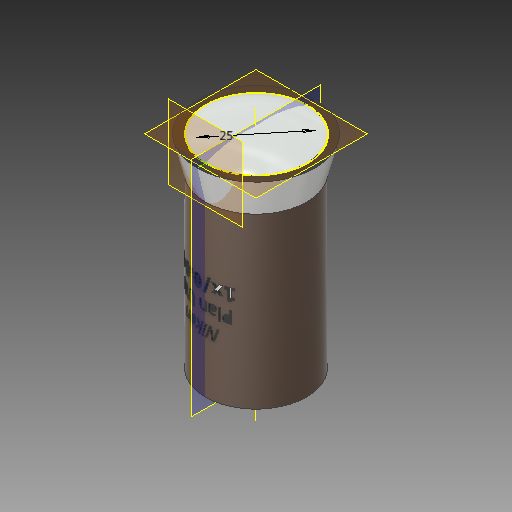
# Autodesk Inventor part: NikonObjective1x
Saved by Autodesk Inventor 2017 (Build 210142000, 142)
## iProperties
Created: 2016-05-20
Part Number: NikonObjective1x
Material: Generic
Document SubType Name: Modeling
Designer: symvoulidis
Density: 1 g/cm^3
Appearance: Smooth - Black
Author: symvoulidis
Autodesk Inventor part; units mm, degrees
ref_plane "YZ Plane" through (0, 0, 0) normal (1, 0, 0) x (0, 1, 0)
ref_plane "XZ Plane" through (0, 0, 0) normal (0, 1, 0) x (-1, 0, 0)
ref_plane "XY Plane" through (0, 0, 0) normal (0, 0, 1) x (1, 0, 0)
sketch "Sketch1" plane through (0, 0, 0) normal (0, 1, 0) x (-1, 0, 0)
  circle A0 centre (0, 0) radius 15
  dimension "d0" = 30
  constraints: 1 centre point, 1 coincident
  measures "d0" diameter of A0
extrude "Extrusion1" add sketch "Sketch1" along normal blind 50
ref_plane "Work Plane1" through (0, 60, 0) normal (0, 1, 0) x (1, 0, 0)
sketch "Sketch2" plane through (0, 60, 0) normal (0, 1, 0) x (1, 0, 0)
  circle A0 centre (0, 0) radius 15 projected
  circle A1 centre (0, 0) radius 12.5
  point P0 (0, -15)
  dimension "d11" = 25
  constraints: 1 centre point, 1 coincident, 1 vertical alignment, 1 other
  measures "d11" diameter of A1
sketch "Sketch3" plane through (0, 60, 0) normal (0, 1, 0) x (1, 0, 0)
  circle A0 centre (0, 0) radius 17.5
  dimension "d4" = 35
  constraints: 1 centre point, 1 coincident
  measures "d4" diameter of A0
loft "Loft1" add profiles "Sketch3" section 2 edges at (15, 50, 0)
ref_plane "Work Plane2" through (0, 60, 15) normal (0, 0, 1) x (1, 0, 0)
sketch "Sketch4" plane through (0, 60, 15) normal (0, 0, 1) x (1, 0, 0)
  line L0 (8.3999, -44.7935) -> (-12.4534, -44.7935) construction
  line L1 (-12.4534, -44.7935) -> (-12.4534, -35.0395) construction
  line L2 (-12.4534, -35.0395) -> (8.3999, -35.0395) construction
  line L3 (8.3999, -35.0395) -> (8.3999, -44.7935) construction
  line L4 (1.1783, -41.1375) -> (1.7002, -41.1375)
  line L5 (1.7002, -41.1375) -> (2.222, -44.1553)
  line L6 (2.222, -44.1553) -> (3.2488, -41.1375)
  line L7 (3.2488, -41.1375) -> (3.6827, -41.1375)
  line L8 (3.6827, -41.1375) -> (2.4943, -44.6375)
  line L9 (2.4943, -44.6375) -> (1.8335, -44.6375)
  line L10 (1.8335, -44.6375) -> (1.3655, -41.8664)
  line L11 (1.3655, -41.8664) -> (0.4238, -44.6375)
  line L12 (0.4238, -44.6375) -> (-0.0101, -44.6375)
  line L13 (-0.0101, -44.6375) -> (1.1783, -41.1375)
  line L14 (0.0523, -41.1375) -> (0.4947, -41.1375)
  line L15 (0.4947, -41.1375) -> (-0.3987, -43.7639)
  line L16 (-0.3987, -43.7639) -> (-0.8412, -43.7639)
  line L17 (-0.8412, -43.7639) -> (0.0523, -41.1375)
  line L18 (-1.0199, -44.2007) -> (-0.5178, -44.2007)
  line L19 (-0.5178, -44.2007) -> (-0.6738, -44.6602)
  line L20 (-0.6738, -44.6602) -> (-1.1759, -44.6602)
  line L21 (-1.1759, -44.6602) -> (-1.0199, -44.2007)
  line L22 (-2.7727, -41.1375) -> (-2.1912, -41.1375)
  line L23 (-2.1912, -41.1375) -> (-1.6467, -42.4053)
  line L24 (-1.6467, -42.4053) -> (-1.4141, -42.2352)
  line L25 (-1.4141, -42.2352) -> (-1.0397, -41.1375)
  line L26 (-1.0397, -41.1375) -> (-0.5972, -41.1375)
  line L27 (-0.5972, -41.1375) -> (-1.8395, -44.7935)
  line L28 (-1.8395, -44.7935) -> (-2.282, -44.7935)
  line L29 (-2.282, -44.7935) -> (-1.5559, -42.6549)
  line L30 (-1.5559, -42.6549) -> (-2.9712, -43.7639)
  line L31 (-2.9712, -43.7639) -> (-3.5215, -43.7639)
  line L32 (-3.5215, -43.7639) -> (-2.0721, -42.6663)
  line L33 (-2.0721, -42.6663) -> (-2.7727, -41.1375)
  spline S0 degree 2 poles (-5.5977, -42.4507) (-5.3736, -41.787) (-4.4887, -41.0638) (-3.9554, -41.0638) knots 0 0 0 1 2 2 2
  spline S1 degree 2 poles (-3.9554, -41.0638) (-3.408, -41.0638) (-3.0365, -41.8097) (-3.252, -42.4507) knots 0 0 0 1 2 2 2
  spline S2 degree 2 poles (-3.252, -42.4507) (-3.4761, -43.1087) (-4.3695, -43.8377) (-4.8999, -43.8377) knots 0 0 0 1 2 2 2
  spline S3 degree 2 poles (-4.8999, -43.8377) (-5.4303, -43.8377) (-5.8217, -43.1116) (-5.5977, -42.4507) knots 0 0 0 1 2 2 2
  spline S4 degree 2 poles (-5.141, -42.4507) (-5.314, -42.9613) (-5.1126, -43.4576) (-4.7695, -43.4576) knots 0 0 0 1 2 2 2
  spline S5 degree 2 poles (-4.7695, -43.4576) (-4.4263, -43.4576) (-3.8817, -42.9613) (-3.7087, -42.4507) knots 0 0 0 1 2 2 2
  spline S6 degree 2 poles (-3.7087, -42.4507) (-3.5413, -41.9544) (-3.7399, -41.4438) (-4.0859, -41.4438) knots 0 0 0 1 2 2 2
  spline S7 degree 2 poles (-4.0859, -41.4438) (-4.4263, -41.4438) (-4.9708, -41.9459) (-5.141, -42.4507) knots 0 0 0 1 2 2 2
  line L34 (-7.6682, -41.1375) -> (-7.2257, -41.1375)
  line L35 (-7.2257, -41.1375) -> (-7.7334, -42.6351)
  spline S8 degree 2 poles (-7.7334, -42.6351) (-7.7958, -42.8166) (-7.8667, -43.1286) (-7.8497, -43.2222) knots 0 0 0 1 2 2 2
  spline S9 degree 2 poles (-7.8497, -43.2222) (-7.8298, -43.3215) (-7.671, -43.4179) (-7.5036, -43.4179) knots 0 0 0 1 2 2 2
  spline S10 degree 2 poles (-7.5036, -43.4179) (-7.3391, -43.4179) (-6.9307, -43.242) (-6.7152, -43.1002) knots 0 0 0 1 2 2 2
  line L36 (-6.7152, -43.1002) -> (-6.0486, -41.1375)
  line L37 (-6.0486, -41.1375) -> (-5.6062, -41.1375)
  line L38 (-5.6062, -41.1375) -> (-6.4996, -43.7639)
  line L39 (-6.4996, -43.7639) -> (-6.9421, -43.7639)
  line L40 (-6.9421, -43.7639) -> (-6.8428, -43.4718)
  spline S11 degree 2 poles (-6.8428, -43.4718) (-7.1009, -43.6505) (-7.549, -43.8377) (-7.7618, -43.8377) knots 0 0 0 1 2 2 2
  spline S12 degree 2 poles (-7.7618, -43.8377) (-8.1503, -43.8377) (-8.4113, -43.3271) (-8.2468, -42.8421) knots 0 0 0 1 2 2 2
  line L41 (-8.2468, -42.8421) -> (-7.6682, -41.1375)
  spline S13 degree 2 poles (4.389, -37.8197) (4.389, -37.5928) (4.5506, -37.1844) (4.6953, -37.0426) knots 0 0 0 1 2 2 2
  spline S14 degree 2 poles (4.6953, -37.0426) (4.8768, -36.8639) (5.3675, -36.6796) (5.7419, -36.6796) knots 0 0 0 1 2 2 2
  line L42 (5.7419, -36.6796) -> (6.1361, -36.6796)
  line L43 (6.1361, -36.6796) -> (6.1361, -35.3749)
  line L44 (6.1361, -35.3749) -> (6.6013, -35.3749)
  line L45 (6.6013, -35.3749) -> (6.6013, -38.8749)
  line L46 (6.6013, -38.8749) -> (5.722, -38.8749)
  spline S15 degree 2 poles (5.722, -38.8749) (5.41, -38.8749) (4.9733, -38.7727) (4.8059, -38.6565) knots 0 0 0 1 2 2 2
  spline S16 degree 2 poles (4.8059, -38.6565) (4.6102, -38.5231) (4.389, -38.1119) (4.389, -37.8197) knots 0 0 0 1 2 2 2
  spline S17 degree 2 poles (4.874, -37.8056) (4.874, -37.9871) (4.9988, -38.2537) (5.1264, -38.3388) knots 0 0 0 1 2 2 2
  spline S18 degree 2 poles (5.1264, -38.3388) (5.237, -38.4125) (5.532, -38.4721) (5.7504, -38.4721) knots 0 0 0 1 2 2 2
  line L47 (5.7504, -38.4721) -> (6.1361, -38.4721)
  line L48 (6.1361, -38.4721) -> (6.1361, -37.0766)
  line L49 (6.1361, -37.0766) -> (5.8185, -37.0766)
  spline S19 degree 2 poles (5.8185, -37.0766) (5.5348, -37.0766) (5.186, -37.1674) (5.0725, -37.2865) knots 0 0 0 1 2 2 2
  spline S20 degree 2 poles (5.0725, -37.2865) (4.9676, -37.3915) (4.874, -37.6382) (4.874, -37.8056) knots 0 0 0 1 2 2 2
  line L50 (3.5296, -35.3749) -> (3.972, -35.3749)
  line L51 (3.972, -35.3749) -> (3.972, -39.0308)
  line L52 (3.972, -39.0308) -> (3.5296, -39.0308)
  line L53 (3.5296, -39.0308) -> (3.5296, -35.3749)
  spline S21 degree 2 poles (1.4165, -35.6528) (1.4704, -35.6131) (1.6519, -35.4713) (1.737, -35.4287) knots 0 0 0 1 2 2 2
  spline S22 degree 2 poles (1.737, -35.4287) (1.8533, -35.3663) (2.0717, -35.3011) (2.2703, -35.3011) knots 0 0 0 1 2 2 2
  spline S23 degree 2 poles (2.2703, -35.3011) (2.4319, -35.3011) (2.7241, -35.4231) (2.8347, -35.5337) knots 0 0 0 1 2 2 2
  spline S24 degree 2 poles (2.8347, -35.5337) (2.9396, -35.6415) (3.0673, -35.9591) (3.0673, -36.135) knots 0 0 0 1 2 2 2
  spline S25 degree 2 poles (3.0673, -36.135) (3.0673, -36.4073) (2.8375, -36.793) (2.5879, -36.9036) knots 0 0 0 1 2 2 2
  spline S26 degree 2 poles (2.5879, -36.9036) (2.3667, -37.0057) (1.7654, -37.0823) (1.4165, -37.1022) knots 0 0 0 1 2 2 2
  line L54 (1.4165, -37.1022) -> (1.4165, -37.1872)
  spline S27 degree 2 poles (1.4165, -37.1872) (1.4165, -37.3404) (1.5101, -37.5304) (1.5952, -37.5843) knots 0 0 0 1 2 2 2
  spline S28 degree 2 poles (1.5952, -37.5843) (1.6803, -37.6382) (1.9242, -37.6723) (2.0547, -37.6723) knots 0 0 0 1 2 2 2
  spline S29 degree 2 poles (2.0547, -37.6723) (2.2079, -37.6723) (2.622, -37.5815) (2.829, -37.4936) knots 0 0 0 1 2 2 2
  line L55 (2.829, -37.4936) -> (2.8545, -37.4936)
  line L56 (2.8545, -37.4936) -> (2.8545, -37.9445)
  spline S30 degree 2 poles (2.8545, -37.9445) (2.7326, -37.9786) (2.2759, -38.0637) (2.0519, -38.0637) knots 0 0 0 1 2 2 2
  spline S31 degree 2 poles (2.0519, -38.0637) (1.7796, -38.0637) (1.408, -37.9786) (1.2605, -37.868) knots 0 0 0 1 2 2 2
  spline S32 degree 2 poles (1.2605, -37.868) (1.1159, -37.7602) (0.9741, -37.417) (0.9741, -37.1702) knots 0 0 0 1 2 2 2
  line L57 (0.9741, -37.1702) -> (0.9741, -35.3749)
  line L58 (0.9741, -35.3749) -> (1.4165, -35.3749)
  line L59 (1.4165, -35.3749) -> (1.4165, -35.6528)
  line L60 (1.4165, -36.0215) -> (1.4165, -36.7505)
  spline S33 degree 2 poles (1.4165, -36.7505) (1.5754, -36.7363) (2.0547, -36.6881) (2.205, -36.6427) knots 0 0 0 1 2 2 2
  spline S34 degree 2 poles (2.205, -36.6427) (2.3809, -36.5888) (2.6106, -36.3647) (2.6106, -36.1662) knots 0 0 0 1 2 2 2
  spline S35 degree 2 poles (2.6106, -36.1662) (2.6106, -35.9393) (2.3553, -35.7095) (2.1114, -35.7095) knots 0 0 0 1 2 2 2
  spline S36 degree 2 poles (2.1114, -35.7095) (1.9044, -35.7095) (1.564, -35.8882) (1.4165, -36.0215) knots 0 0 0 1 2 2 2
  line L61 (-1.7091, -35.3749) -> (-1.2666, -35.3749)
  line L62 (-1.2666, -35.3749) -> (-1.2666, -36.8724)
  spline S37 degree 2 poles (-1.2666, -36.8724) (-1.2666, -37.0539) (-1.2326, -37.3659) (-1.1815, -37.4595) knots 0 0 0 1 2 2 2
  spline S38 degree 2 poles (-1.1815, -37.4595) (-1.1276, -37.5588) (-0.9348, -37.6552) (-0.7703, -37.6552) knots 0 0 0 1 2 2 2
  spline S39 degree 2 poles (-0.7703, -37.6552) (-0.6058, -37.6552) (-0.2569, -37.4794) (-0.0895, -37.3376) knots 0 0 0 1 2 2 2
  line L63 (-0.0895, -37.3376) -> (-0.0895, -35.3749)
  line L64 (-0.0895, -35.3749) -> (0.3529, -35.3749)
  line L65 (0.3529, -35.3749) -> (0.3529, -38.0013)
  line L66 (0.3529, -38.0013) -> (-0.0895, -38.0013)
  line L67 (-0.0895, -38.0013) -> (-0.0895, -37.7091)
  spline S40 degree 2 poles (-0.0895, -37.7091) (-0.2881, -37.8878) (-0.671, -38.075) (-0.8865, -38.075) knots 0 0 0 1 2 2 2
  spline S41 degree 2 poles (-0.8865, -38.075) (-1.2723, -38.075) (-1.7091, -37.5645) (-1.7091, -37.0795) knots 0 0 0 1 2 2 2
  line L68 (-1.7091, -37.0795) -> (-1.7091, -35.3749)
  spline S42 degree 2 poles (-5.09, -35.3011) (-4.7808, -35.3011) (-4.3213, -35.4628) (-4.1596, -35.6244) knots 0 0 0 1 2 2 2
  spline S43 degree 2 poles (-4.1596, -35.6244) (-3.9753, -35.806) (-3.825, -36.3165) (-3.825, -36.6909) knots 0 0 0 1 2 2 2
  line L69 (-3.825, -36.6909) -> (-3.825, -38.8749)
  line L70 (-3.825, -38.8749) -> (-4.2901, -38.8749)
  line L71 (-4.2901, -38.8749) -> (-4.2901, -36.6909)
  spline S44 degree 2 poles (-4.2901, -36.6909) (-4.2901, -36.447) (-4.3525, -36.118) (-4.4404, -35.9847) knots 0 0 0 1 2 2 2
  spline S45 degree 2 poles (-4.4404, -35.9847) (-4.534, -35.8428) (-4.8574, -35.6982) (-5.09, -35.6982) knots 0 0 0 1 2 2 2
  spline S46 degree 2 poles (-5.09, -35.6982) (-5.3083, -35.6982) (-5.6487, -35.8428) (-5.7423, -35.9847) knots 0 0 0 1 2 2 2
  spline S47 degree 2 poles (-5.7423, -35.9847) (-5.8302, -36.118) (-5.8926, -36.4441) (-5.8926, -36.6796) knots 0 0 0 1 2 2 2
  line L72 (-5.8926, -36.6796) -> (-5.8926, -38.8749)
  line L73 (-5.8926, -38.8749) -> (-6.3578, -38.8749)
  line L74 (-6.3578, -38.8749) -> (-6.3578, -36.6909)
  spline S48 degree 2 poles (-6.3578, -36.6909) (-6.3578, -36.325) (-6.2103, -35.8031) (-6.0231, -35.6244) knots 0 0 0 1 2 2 2
  spline S49 degree 2 poles (-6.0231, -35.6244) (-5.8558, -35.4599) (-5.4133, -35.3011) (-5.09, -35.3011) knots 0 0 0 1 2 2 2
  line L75 (-10.9469, -38.8749) -> (-10.0677, -35.3749)
  line L76 (-10.0677, -35.3749) -> (-9.5458, -35.3749)
  line L77 (-9.5458, -35.3749) -> (-8.8339, -38.2792)
  line L78 (-8.8339, -38.2792) -> (-8.1418, -35.3749)
  line L79 (-8.1418, -35.3749) -> (-7.6256, -35.3749)
  line L80 (-7.6256, -35.3749) -> (-6.7322, -38.8749)
  line L81 (-6.7322, -38.8749) -> (-7.2115, -38.8749)
  line L82 (-7.2115, -38.8749) -> (-7.9149, -35.9733)
  line L83 (-7.9149, -35.9733) -> (-8.6126, -38.8749)
  line L84 (-8.6126, -38.8749) -> (-9.0863, -38.8749)
  line L85 (-9.0863, -38.8749) -> (-9.7897, -35.9393)
  line L86 (-9.7897, -35.9393) -> (-10.4903, -38.8749)
  line L87 (-10.4903, -38.8749) -> (-10.9469, -38.8749)
  line L88 (4.9293, -29.6122) -> (7.2409, -29.6122)
  line L89 (7.2409, -29.6122) -> (7.2409, -30.222)
  line L90 (7.2409, -30.222) -> (6.5034, -30.222)
  line L91 (6.5034, -30.222) -> (6.5034, -32.0741)
  line L92 (6.5034, -32.0741) -> (7.2409, -32.0741)
  line L93 (7.2409, -32.0741) -> (7.2409, -32.6442)
  spline S50 degree 2 poles (7.2409, -32.6442) (7.0792, -32.6442) (6.7587, -32.6867) (6.6623, -32.7321) knots 0 0 0 1 2 2 2
  spline S51 degree 2 poles (6.6623, -32.7321) (6.5517, -32.7889) (6.4269, -32.9789) (6.4155, -33.1207) knots 0 0 0 1 2 2 2
  line L94 (6.4155, -33.1207) -> (5.6497, -33.1207)
  line L95 (5.6497, -33.1207) -> (5.6497, -30.222)
  line L96 (5.6497, -30.222) -> (4.9293, -30.222)
  line L97 (4.9293, -30.222) -> (4.9293, -29.6122)
  line L98 (1.7158, -29.6122) -> (2.6801, -29.6122)
  line L99 (2.6801, -29.6122) -> (3.1821, -30.3695)
  line L100 (3.1821, -30.3695) -> (3.6983, -29.6122)
  line L101 (3.6983, -29.6122) -> (4.6428, -29.6122)
  line L102 (4.6428, -29.6122) -> (3.67, -30.9339)
  line L103 (3.67, -30.9339) -> (4.6258, -32.2528)
  line L104 (4.6258, -32.2528) -> (3.6615, -32.2528)
  line L105 (3.6615, -32.2528) -> (3.1679, -31.5097)
  line L106 (3.1679, -31.5097) -> (2.6716, -32.2528)
  line L107 (2.6716, -32.2528) -> (1.7271, -32.2528)
  line L108 (1.7271, -32.2528) -> (2.6829, -30.9538)
  line L109 (2.6829, -30.9538) -> (1.7158, -29.6122)
  line L110 (-0.6214, -33.2682) -> (0.7713, -28.8521)
  line L111 (0.7713, -28.8521) -> (1.4463, -28.8521)
  line L112 (1.4463, -28.8521) -> (0.0565, -33.2682)
  line L113 (0.0565, -33.2682) -> (-0.6214, -33.2682)
  spline S52 degree 2 poles (-3.9342, -31.3622) (-3.9342, -30.9084) (-3.7895, -30.2277) (-3.6278, -29.9979) knots 0 0 0 1 2 2 2
  spline S53 degree 2 poles (-3.6278, -29.9979) (-3.469, -29.771) (-2.9556, -29.5384) (-2.5869, -29.5384) knots 0 0 0 1 2 2 2
  spline S54 degree 2 poles (-2.5869, -29.5384) (-2.2154, -29.5384) (-1.7048, -29.771) (-1.5432, -30.0036) knots 0 0 0 1 2 2 2
  spline S55 degree 2 poles (-1.5432, -30.0036) (-1.3815, -30.2333) (-1.2368, -30.9084) (-1.2368, -31.3622) knots 0 0 0 1 2 2 2
  spline S56 degree 2 poles (-1.2368, -31.3622) (-1.2368, -31.8273) (-1.3815, -32.4854) (-1.546, -32.7236) knots 0 0 0 1 2 2 2
  spline S57 degree 2 poles (-1.546, -32.7236) (-1.7105, -32.9562) (-2.2295, -33.1831) (-2.5869, -33.1831) knots 0 0 0 1 2 2 2
  spline S58 degree 2 poles (-2.5869, -33.1831) (-2.9641, -33.1831) (-3.469, -32.9449) (-3.6307, -32.7094) knots 0 0 0 1 2 2 2
  spline S59 degree 2 poles (-3.6307, -32.7094) (-3.7895, -32.4797) (-3.9342, -31.8018) (-3.9342, -31.3622) knots 0 0 0 1 2 2 2
  spline S60 degree 2 poles (-3.0521, -31.3622) (-3.0521, -32.0117) (-2.8393, -32.5364) (-2.5869, -32.5364) knots 0 0 0 1 2 2 2
  spline S61 degree 2 poles (-2.5869, -32.5364) (-2.3345, -32.5364) (-2.1189, -32.0117) (-2.1189, -31.3594) knots 0 0 0 1 2 2 2
  spline S62 degree 2 poles (-2.1189, -31.3594) (-2.1189, -30.7184) (-2.3345, -30.1851) (-2.5869, -30.1851) knots 0 0 0 1 2 2 2
  spline S63 degree 2 poles (-2.5869, -30.1851) (-2.8365, -30.1851) (-3.0521, -30.7184) (-3.0521, -31.3622) knots 0 0 0 1 2 2 2
  line L114 (-5.2842, -29.6122) -> (-4.4532, -29.6122)
  line L115 (-4.4532, -29.6122) -> (-4.4532, -30.5368)
  line L116 (-4.4532, -30.5368) -> (-5.2842, -30.5368)
  line L117 (-5.2842, -30.5368) -> (-5.2842, -29.6122)
  spline S64 degree 2 poles (-8.5034, -31.3622) (-8.5034, -30.9084) (-8.3588, -30.2277) (-8.1971, -29.9979) knots 0 0 0 1 2 2 2
  spline S65 degree 2 poles (-8.1971, -29.9979) (-8.0383, -29.771) (-7.5249, -29.5384) (-7.1562, -29.5384) knots 0 0 0 1 2 2 2
  spline S66 degree 2 poles (-7.1562, -29.5384) (-6.7846, -29.5384) (-6.2741, -29.771) (-6.1124, -30.0036) knots 0 0 0 1 2 2 2
  spline S67 degree 2 poles (-6.1124, -30.0036) (-5.9508, -30.2333) (-5.8061, -30.9084) (-5.8061, -31.3622) knots 0 0 0 1 2 2 2
  spline S68 degree 2 poles (-5.8061, -31.3622) (-5.8061, -31.8273) (-5.9508, -32.4854) (-6.1153, -32.7236) knots 0 0 0 1 2 2 2
  spline S69 degree 2 poles (-6.1153, -32.7236) (-6.2798, -32.9562) (-6.7988, -33.1831) (-7.1562, -33.1831) knots 0 0 0 1 2 2 2
  spline S70 degree 2 poles (-7.1562, -33.1831) (-7.5334, -33.1831) (-8.0383, -32.9449) (-8.2, -32.7094) knots 0 0 0 1 2 2 2
  spline S71 degree 2 poles (-8.2, -32.7094) (-8.3588, -32.4797) (-8.5034, -31.8018) (-8.5034, -31.3622) knots 0 0 0 1 2 2 2
  spline S72 degree 2 poles (-7.6214, -31.3622) (-7.6214, -32.0117) (-7.4086, -32.5364) (-7.1562, -32.5364) knots 0 0 0 1 2 2 2
  spline S73 degree 2 poles (-7.1562, -32.5364) (-6.9038, -32.5364) (-6.6882, -32.0117) (-6.6882, -31.3594) knots 0 0 0 1 2 2 2
  spline S74 degree 2 poles (-6.6882, -31.3594) (-6.6882, -30.7184) (-6.9038, -30.1851) (-7.1562, -30.1851) knots 0 0 0 1 2 2 2
  spline S75 degree 2 poles (-7.1562, -30.1851) (-7.4058, -30.1851) (-7.6214, -30.7184) (-7.6214, -31.3622) knots 0 0 0 1 2 2 2
  line L118 (-11.6574, -30.429) -> (-11.1838, -30.429)
  line L119 (-11.1838, -30.429) -> (-11.1838, -29.6037)
  line L120 (-11.1838, -29.6037) -> (-10.3357, -29.6037)
  line L121 (-10.3357, -29.6037) -> (-10.3357, -30.429)
  line L122 (-10.3357, -30.429) -> (-8.7927, -30.429)
  line L123 (-8.7927, -30.429) -> (-8.7927, -31.0814)
  line L124 (-8.7927, -31.0814) -> (-10.3073, -33.1122)
  line L125 (-10.3073, -33.1122) -> (-11.1838, -33.1122)
  line L126 (-11.1838, -33.1122) -> (-11.1838, -31.0587)
  line L127 (-11.1838, -31.0587) -> (-11.6574, -31.0587)
  line L128 (-11.6574, -31.0587) -> (-11.6574, -30.429)
  line L129 (-10.3357, -31.0587) -> (-10.3357, -32.25)
  line L130 (-10.3357, -32.25) -> (-9.4479, -31.0587)
  line L131 (-9.4479, -31.0587) -> (-10.3357, -31.0587)
  point P0 (0, -60)
  constraints: 2 other
emboss "Emboss1" sketch "Sketch4" operation cut depth 1 direction (0, 0, -1) wrap yes faces at (-14.9514, 16.6667, -1.207)
ref_plane "Work Plane3" through (0, 0, 0) normal (-1, 0, 0) x (0, -1, 0)
sketch "Sketch5" plane through (0, 0, 0) normal (-1, 0, 0) x (0, -1, 0)
  line L0 (-60, -17.5) -> (-60, 17.5) projected
  line L1 (-60, 0) -> (-60, -15)
  line L2 (-60, -15) -> (-60, 0)
  arc A0 (-62.0953, 0) -> (-60, -15) centre (-31.8408, -3.4203) ccw
  line L3 (-62.0953, 0) -> (-60, 0)
  line L4 (-50, 15) -> (-50, -15) projected
  line L5 (-60, -15) -> (-60, 0)
  line L6 (-75.6514, 0) -> (12.6086, 0) projected
  point P0 (0, 0)
  dimension "d13" = 15
  constraints: 8 end point, 2 collinear, 2 point on circle, 1 centre point, 1 midpoint, 1 perpendicular, 1 point on line
  measures "d13" distance of L1.start L1.end
revolve "Revolution1" add sketch "Sketch5" angle 360 about axis through (0, 0, 0) along (0, -1, 0)
body "Solid1"
